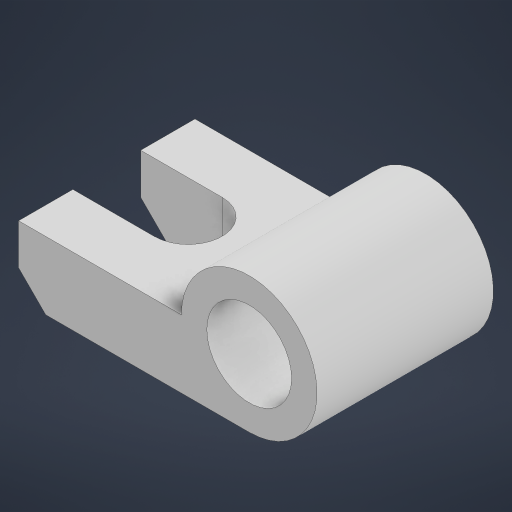
# Autodesk Inventor part: Część21
Saved by Autodesk Inventor 2023 (Build 270158000, 158)
## iProperties
Created: 2023-05-08
Part Number: Część21
Material: Ogólny
Document SubType Name: Modeling
Designer: Adam
Density: 1 g/cm^3
Appearance: Domyślna
Author: Adam
Autodesk Inventor part; units mm, degrees
ref_plane "YZ Plane" through (0, 0, 0) normal (1, 0, 0) x (0, 1, 0)
ref_plane "XZ Plane" through (0, 0, 0) normal (0, 1, 0) x (-1, 0, 0)
ref_plane "XY Plane" through (0, 0, 0) normal (0, 0, 1) x (1, 0, 0)
sketch "Szkic1" plane through (0, 0, 0) normal (0, 0, 1) x (1, 0, 0)
  line L0 (0, 0) -> (34, 0)
  line L1 (34, 0) -> (34, 10)
  line L2 (34, 10) -> (0, 10)
  line L3 (0, 10) -> (0, 0)
  circle A0 centre (34, 10) radius 10
  point P0 (24, 10)
  dimension "d0" = 34
  dimension "d1" = 10
  dimension "d2" = 20
  constraints: 8 end point, 2 parallel, 1 centre point, 1 coincident, 1 horizontal, 1 perpendicular
  measures "d0" distance of L2.end L1.end
  measures "d1" distance of L1.end L0.end
  measures "d2" diameter of A0
extrude "Wyciągnięcie proste1" add sketch "Szkic1" along normal mid plane 26
chamfer "Faza1" distance 4 angle 45 1 edges at (0, 0, 0)
sketch "Szkic2" plane through (0, 0, 13) normal (0, 0, 1) x (1, 0, 0)
  arc A0 (34, 0) -> (24, 10) centre (34, 10) ccw projected
  point P0 (0, 0)
  constraints: 1 coincident
hole "Otwór1" at (34, 10, 13) direction (0, 0, -1) diameter 12.5 end through all
sketch "Szkic3" plane through (0, 10, 13) normal (0, 1, 0) x (1, 0, 0)
  line L0 (0, 18) -> (12, 18)
  line L1 (12, 18) -> (12, 8)
  line L2 (12, 8) -> (0, 8)
  line L3 (0, 8) -> (0, 18)
  circle A0 centre (12, 13) radius 5
  point P0 (0, 13)
  constraints: 8 end point, 2 parallel, 1 centre point, 1 horizontal, 1 midpoint, 1 perpendicular
extrude "Wyciągnięcie proste2" cut sketch "Szkic3" against normal through all
